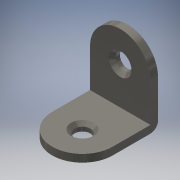
# Autodesk Inventor part: MellewellCornerBrace
Saved by Autodesk Inventor 2018 (Build 220112000, 112)
## iProperties
Created: 2017-12-21
Part Number: MellewellCornerBrace
Material: Generic
Document SubType Name: Modeling
Designer: jklei
Density: 1 g/cm^3
Appearance: Default
Author: jklei
Autodesk Inventor part; units mm, degrees
ref_plane "YZ Plane" through (0, 0, 0) normal (1, 0, 0) x (0, 1, 0)
ref_plane "XZ Plane" through (0, 0, 0) normal (0, 1, 0) x (-1, 0, 0)
ref_plane "XY Plane" through (0, 0, 0) normal (0, 0, 1) x (1, 0, 0)
sketch "Sketch1" plane through (0, 0, 0) normal (1, 0, 0) x (0, 1, 0)
  line L0 (0, 0) -> (2, 0)
  line L1 (0, 0) -> (0, -18)
  line L2 (2, -20) -> (20, -20)
  line L3 (20, -20) -> (20, -18)
  line L4 (20, -18) -> (2, -18)
  line L5 (2, 0) -> (2, -18)
  arc A0 (0, -18) -> (2, -20) centre (2, -18) ccw
  point P0 (0, -20)
  dimension "d0" = 2
  dimension "d1" = 20
  dimension "d2" = 20
  dimension "d3" = 2
  dimension "d4" = 2
  constraints: 12 end point, 3 perpendicular, 2 point on circle, 2 point on line, 2 tangent, 2 vertical, 1 centre point, 1 horizontal
  measures "d0" distance of L0.start L0.end
  measures "d1" distance of L0.start point (0, -20)
  measures "d2" distance of point (0, -20) L2.end
  measures "d3" distance of L2.end L3.end
  measures "d4" radius of A0
extrude "Extrusion1" add sketch "Sketch1" along normal blind 16
fillet "Fillet2" radius 8 4 edges at (16, 20, -19) (0, 20, -19) (0, 1, 0) (16, 1, 0)
sketch "Sketch2" plane through (0, 2, -18) normal (0, 0, 1) x (1, 0, 0)
  line L0 (0, 0) -> (0, 10) projected
  line L1 (0, 0) -> (16, 0) projected
  line L2 (16, 10) -> (16, 0) projected
  arc A0 (16, 10) -> (0, 10) centre (8, 10) ccw projected
  line L3 (0, 0) -> (16, 0) projected
  point P0 (0, -2)
hole "Hole1" at (8, 12, -18) direction (0, 0, -1) diameter 4.2 end through all countersink diameter 6 countersink angle 90
sketch "Sketch4" plane through (0, 2, -18) normal (0, 1, 0) x (1, 0, 0)
  arc A0 (0, -10) -> (16, -10) centre (8, -10) ccw projected
  line L0 (16, 0) -> (16, -10) projected
  line L1 (0, 0) -> (16, 0) projected
  line L2 (0, -10) -> (0, 0) projected
  point P0 (0, -18)
hole "Hole3" at (8, 2, -8) direction (0, -1, 0) diameter 4.2 end through all countersink diameter 6 countersink angle 90
body "Solid1"
